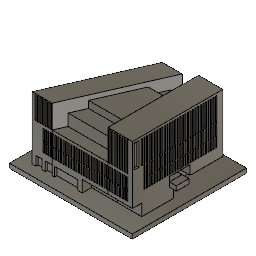
Marshgate v15 (Autodesk Fusion 360 design; units mm, degrees)
Autodesk Fusion 360 part; units mm, degrees
(part 1 of 2)
sketch "Sketch1" plane through (0, 0, 0) normal (0, 0, 1) x (1, 0, 0)
  line L0 (45.5671, 66.2073) -> (45.5671, 27.2073)
  line L1 (45.5671, 27.2073) -> (2.2671, 27.2073)
  line L2 (45.5671, 66.2073) -> (19.3671, 66.2073)
  line L3 (19.3671, 66.2073) -> (2.2671, 27.2073)
  line L4 (45.5671, 66.2073) -> (35, 66.2073)
  line L5 (35, 27.2073) -> (35, 66.2073)
  line L6 (28.0686, 66.2073) -> (10.9686, 27.2073)
  line L7 (13.0575, 31.9714) -> (35, 31.9714)
  line L8 (15.7468, 38.1049) -> (35, 38.1049)
  line L9 (23.5655, 55.9369) -> (35, 55.9369)
  line L10 (26.4855, 62.5965) -> (35, 62.5965)
  line L11 (42, 62) -> (26, 69)
  line L12 (26, 69) -> (24, 61)
  line L13 (24, 61) -> (42, 62)
  line L14 (50.0207, 22.6472) -> (-2.9555, 22.6472)
  line L15 (-2.9555, 22.6472) -> (-2.9555, 71.9468)
  line L16 (-2.9555, 71.9468) -> (50.0207, 71.9468)
  line L17 (50.0207, 71.9468) -> (50.0207, 22.6472)
  line L18 (-2.9555, 33.4173) -> (13.9382, 71.9468)
  dimension "d1" = 39
  dimension "d2" = 43.3
  dimension "d3" = 26.2
  constraint vertical L0
  constraint perpendicular L0 L1
  constraint perpendicular L0 L2
  constraint coincident L2 L4.end
  constraint coincident L1 L5.start
  constraint perpendicular L2 L5
  constraint coincident L2 L6.start
  constraint coincident L1 L6.end
  constraint parallel L3 L6
  constraint coincident L6 L7.start
  constraint coincident L5 L7.end
  constraint perpendicular L5 L7
  constraint coincident L6 L8.start
  constraint coincident L5 L8.end
  constraint perpendicular L5 L8
  constraint coincident L6 L9.start
  constraint coincident L5 L9.end
  constraint perpendicular L5 L9
  constraint coincident L6 L10.start
  constraint coincident L5 L10.end
  constraint perpendicular L5 L10
  constraint horizontal L14
  constraint vertical L15
  constraint horizontal L16
  constraint vertical L17
  constraint coincident L15 L18.start
  constraint coincident L16 L18.end
  constraint parallel L3 L18
  measures "d1" distance of L0.start L0.end
  measures "d2" distance of L0.end L1.end
  measures "d3" distance of L0.start L2.end
extrude "Extrude1" add sketch "Sketch1" along normal blind 30 contours L0 L1 L2 L4 L5 L11 L13 | L5 L11 L13 makes body 1
extrude "Extrude2" add sketch "Sketch1" along normal blind 27 separate body contours L1 L2 L3 L6 L12 L13 | L2 L6 L12 L13 makes body 2
extrude "Extrude3" add sketch "Sketch1" along normal blind 25 separate body contours L5 L6 L8 L9 makes body 3
extrude "Extrude4" add sketch "Sketch1" along normal blind 22 separate body contours L5 L6 L7 L8 makes body 4
extrude "Extrude5" add sketch "Sketch1" along normal blind 17 separate body contours L1 L5 L6 L7 makes body 5
extrude "Extrude6" add sketch "Sketch1" along normal blind 22 separate body contours L5 L6 L10 L13 | L5 L6 L9 L13 makes body 6
extrude "Extrude7" add sketch "Sketch1" along normal blind 10 separate body contours L2 L5 L11 | L2 L5 L6 L10 L11 makes body 7
sketch "Sketch2" plane through (0, 27.2073, 0) normal (0, -1, 0) x (1, 0, 0)
  line L0 (10.9686, 0) -> (35, 0)
  line L1 (35, 0) -> (35, 17)
  line L2 (35, 17) -> (10.9686, 17)
  line L3 (10.9686, 17) -> (10.9686, 0)
  line L4 (35, 10) -> (28.0686, 10)
  line L5 (2.2671, 0) -> (10.9686, 0)
  line L6 (10.9686, 0) -> (10.9686, 27)
  line L7 (10.9686, 27) -> (2.2671, 27)
  line L8 (2.2671, 27) -> (2.2671, 0)
  line L9 (35, 0) -> (45.5671, 0)
  line L10 (45.5671, 0) -> (45.5671, 30)
  line L11 (45.5671, 30) -> (35, 30)
  line L12 (35, 30) -> (35, 0)
  line L13 (2.2671, 0) -> (45.5671, 0)
  line L14 (45.5671, 0) -> (45.5671, 5.0322)
  line L15 (45.5671, 5.0322) -> (2.2671, 5.0322)
  line L16 (2.2671, 5.0322) -> (2.2671, 0)
  line L17 (23.9171, 5.0322) -> (35, 5.0322)
  line L18 (35, 5.0322) -> (35, 0)
  line L19 (35, 0) -> (23.9171, 0)
  line L20 (23.9171, 0) -> (23.9171, 5.0322)
  line L21 (22, 4) -> (12, 4)
  line L22 (12, 4) -> (12, 0)
  line L23 (12, 0) -> (22, 0)
  line L24 (22, 0) -> (22, 4)
  line L25 (4, 4) -> (6.6179, 4)
  line L26 (6.6179, 4) -> (6.6179, 0)
  line L27 (6.6179, 0) -> (4, 0)
  line L28 (4, 0) -> (4, 4)
  line L29 (8, 4) -> (10.9686, 4)
  line L30 (10.9686, 4) -> (10.9686, 0)
  line L31 (10.9686, 0) -> (8, 0)
  line L32 (8, 0) -> (8, 4)
  line L33 (24.9513, 10.7057) -> (24.4513, 10.7057)
  line L34 (27.7625, 10.7057) -> (27.7625, 15.6501)
  line L35 (23.3549, 10.3545) -> (23.8549, 10.3545)
  line L36 (26.6587, 10.7057) -> (26.6587, 15.6501)
  line L37 (24.4513, 10.7057) -> (24.4513, 15.6501)
  line L38 (17.2292, 6.6128) -> (16.7292, 6.6128)
  line L39 (17.8291, 15.6501) -> (18.3291, 15.6501)
  line L40 (18.3291, 15.6501) -> (18.3291, 10.7057)
  line L41 (21.6402, 15.6501) -> (21.6402, 10.7057)
  line L42 (17.8334, 10.3545) -> (18.3334, 10.3545)
  line L43 (20.042, 10.3545) -> (20.542, 10.3545)
  line L44 (22.2439, 15.6501) -> (22.7439, 15.6501)
  line L45 (21.1402, 10.7057) -> (21.1402, 15.6501)
  line L46 (18.9377, 10.3545) -> (19.4377, 10.3545)
  line L47 (18.9328, 15.6501) -> (19.4328, 15.6501)
  line L48 (21.1463, 10.3545) -> (21.6463, 10.3545)
  line L49 (22.7439, 10.7057) -> (22.2439, 10.7057)
  line L50 (19.4328, 10.7057) -> (18.9328, 10.7057)
  line L51 (21.6402, 10.7057) -> (21.1402, 10.7057)
  line L52 (20.0365, 15.6501) -> (20.5365, 15.6501)
  line L53 (23.8476, 15.6501) -> (23.8476, 10.7057)
  line L54 (24.4592, 10.3545) -> (24.9592, 10.3545)
  line L55 (23.3476, 15.6501) -> (23.8476, 15.6501)
  line L56 (27.1587, 10.7057) -> (26.6587, 10.7057)
  line L57 (25.5634, 10.3545) -> (26.0634, 10.3545)
  line L58 (25.555, 15.6501) -> (26.055, 15.6501)
  line L59 (23.3476, 10.7057) -> (23.3476, 15.6501)
  line L60 (12.812, 6.6128) -> (12.312, 6.6128)
  line L61 (24.9592, 6.6128) -> (24.4592, 6.6128)
  line L62 (20.542, 6.6128) -> (20.042, 6.6128)
  line L63 (21.6463, 6.6128) -> (21.1463, 6.6128)
  line L64 (26.0634, 6.6128) -> (25.5634, 6.6128)
  line L65 (18.3334, 6.6128) -> (17.8334, 6.6128)
  line L66 (23.8476, 10.7057) -> (23.3476, 10.7057)
  line L67 (26.6677, 10.3545) -> (27.1677, 10.3545)
  line L68 (26.6587, 15.6501) -> (27.1587, 15.6501)
  line L69 (26.055, 15.6501) -> (26.055, 10.7057)
  line L70 (27.1587, 15.6501) -> (27.1587, 10.7057)
  line L71 (26.055, 10.7057) -> (25.555, 10.7057)
  line L72 (24.9513, 15.6501) -> (24.9513, 10.7057)
  line L73 (24.4513, 15.6501) -> (24.9513, 15.6501)
  line L74 (25.555, 10.7057) -> (25.555, 15.6501)
  line L75 (16.1217, 15.6501) -> (16.1217, 10.7057)
  line L76 (11.2077, 10.3545) -> (11.7077, 10.3545)
  line L77 (13.9143, 15.6501) -> (13.9143, 10.7057)
  line L78 (11.7069, 15.6501) -> (11.7069, 10.7057)
  line L79 (17.2254, 15.6501) -> (17.2254, 10.7057)
  line L80 (15.6249, 10.3545) -> (16.1249, 10.3545)
  line L81 (22.7506, 6.6128) -> (22.2506, 6.6128)
  line L82 (19.4377, 6.6128) -> (18.9377, 6.6128)
  line L83 (11.7077, 6.6128) -> (11.2077, 6.6128)
  line L84 (27.1677, 6.6128) -> (26.6677, 6.6128)
  line L85 (16.1249, 6.6128) -> (15.6249, 6.6128)
  line L86 (23.8549, 6.6128) -> (23.3549, 6.6128)
  line L87 (15.0206, 6.6128) -> (14.5206, 6.6128)
  line L88 (10.6034, 6.6128) -> (10.1034, 6.6128)
  line L89 (13.9163, 6.6128) -> (13.4163, 6.6128)
  line L90 (23.3549, 6.6128) -> (23.3549, 10.3545)
  line L91 (16.1249, 10.3545) -> (16.1249, 6.6128)
  line L92 (10.6034, 10.3545) -> (10.6034, 6.6128)
  line L93 (16.7292, 6.6128) -> (16.7292, 10.3545)
  line L94 (27.772, 10.3545) -> (28.272, 10.3545)
  line L95 (15.0206, 10.3545) -> (15.0206, 6.6128)
  line L96 (24.4592, 6.6128) -> (24.4592, 10.3545)
  line L97 (27.7625, 15.6501) -> (28.2625, 15.6501)
  line L98 (22.2506, 6.6128) -> (22.2506, 10.3545)
  line L99 (26.0634, 10.3545) -> (26.0634, 6.6128)
  line L100 (28.2625, 10.7057) -> (27.7625, 10.7057)
  line L101 (21.6463, 10.3545) -> (21.6463, 6.6128)
  line L102 (22.7506, 10.3545) -> (22.7506, 6.6128)
  line L103 (20.542, 10.3545) -> (20.542, 6.6128)
  line L104 (13.4163, 6.6128) -> (13.4163, 10.3545)
  line L105 (18.9377, 6.6128) -> (18.9377, 10.3545)
  line L106 (19.4377, 10.3545) -> (19.4377, 6.6128)
  line L107 (27.772, 6.6128) -> (27.772, 10.3545)
  line L108 (25.5634, 6.6128) -> (25.5634, 10.3545)
  line L109 (18.3334, 10.3545) -> (18.3334, 6.6128)
  line L110 (21.1463, 6.6128) -> (21.1463, 10.3545)
  line L111 (20.5365, 10.7057) -> (20.0365, 10.7057)
  line L112 (20.5365, 15.6501) -> (20.5365, 10.7057)
  line L113 (18.9328, 10.7057) -> (18.9328, 15.6501)
  line L114 (22.2439, 10.7057) -> (22.2439, 15.6501)
  line L115 (18.3291, 10.7057) -> (17.8291, 10.7057)
  line L116 (21.1402, 15.6501) -> (21.6402, 15.6501)
  line L117 (20.0365, 10.7057) -> (20.0365, 15.6501)
  line L118 (19.4328, 15.6501) -> (19.4328, 10.7057)
  line L119 (22.2506, 10.3545) -> (22.7506, 10.3545)
  line L120 (22.7439, 15.6501) -> (22.7439, 10.7057)
  line L121 (17.8291, 10.7057) -> (17.8291, 15.6501)
  line L122 (13.4163, 10.3545) -> (13.9163, 10.3545)
  line L123 (16.7254, 15.6501) -> (17.2254, 15.6501)
  line L124 (16.7254, 10.7057) -> (16.7254, 15.6501)
  line L125 (12.312, 10.3545) -> (12.812, 10.3545)
  line L126 (11.2069, 15.6501) -> (11.7069, 15.6501)
  line L127 (14.5206, 10.3545) -> (15.0206, 10.3545)
  line L128 (17.2254, 10.7057) -> (16.7254, 10.7057)
  line L129 (15.018, 15.6501) -> (15.018, 10.7057)
  line L130 (13.4143, 15.6501) -> (13.9143, 15.6501)
  line L131 (13.9143, 10.7057) -> (13.4143, 10.7057)
  line L132 (11.7069, 10.7057) -> (11.2069, 10.7057)
  line L133 (10.6034, 15.6501) -> (10.6034, 10.7057)
  line L134 (16.7292, 10.3545) -> (17.2292, 10.3545)
  line L135 (12.8106, 10.7057) -> (12.3106, 10.7057)
  line L136 (16.1217, 10.7057) -> (15.6217, 10.7057)
  line L137 (14.518, 15.6501) -> (15.018, 15.6501)
  line L138 (10.1034, 10.3545) -> (10.6034, 10.3545)
  line L139 (27.1677, 10.3545) -> (27.1677, 6.6128)
  line L140 (24.9592, 10.3545) -> (24.9592, 6.6128)
  line L141 (10.1034, 6.6128) -> (10.1034, 10.3545)
  line L142 (12.812, 10.3545) -> (12.812, 6.6128)
  line L143 (11.2077, 6.6128) -> (11.2077, 10.3545)
  line L144 (11.7077, 10.3545) -> (11.7077, 6.6128)
  line L145 (26.6677, 6.6128) -> (26.6677, 10.3545)
  line L146 (15.6249, 6.6128) -> (15.6249, 10.3545)
  line L147 (23.8549, 10.3545) -> (23.8549, 6.6128)
  line L148 (20.042, 6.6128) -> (20.042, 10.3545)
  line L149 (17.8334, 6.6128) -> (17.8334, 10.3545)
  line L150 (17.2292, 10.3545) -> (17.2292, 6.6128)
  line L151 (14.5206, 6.6128) -> (14.5206, 10.3545)
  line L152 (13.9163, 10.3545) -> (13.9163, 6.6128)
  line L153 (12.312, 6.6128) -> (12.312, 10.3545)
  line L154 (11.2069, 10.7057) -> (11.2069, 15.6501)
  line L155 (10.1034, 10.7057) -> (10.1034, 15.6501)
  line L156 (15.6217, 15.6501) -> (16.1217, 15.6501)
  line L157 (15.018, 10.7057) -> (14.518, 10.7057)
  line L158 (10.6034, 10.7057) -> (10.1034, 10.7057)
  line L159 (14.518, 10.7057) -> (14.518, 15.6501)
  line L160 (12.3106, 10.7057) -> (12.3106, 15.6501)
  line L161 (13.4143, 10.7057) -> (13.4143, 15.6501)
  line L162 (10.1034, 15.6501) -> (10.6034, 15.6501)
  line L163 (15.6217, 10.7057) -> (15.6217, 15.6501)
  line L164 (12.3106, 15.6501) -> (12.8106, 15.6501)
  line L165 (12.8106, 15.6501) -> (12.8106, 10.7057)
  line L166 (38.8149, 6.6128) -> (38.8149, 10.3545)
  line L167 (31.0736, 15.6501) -> (31.5736, 15.6501)
  line L168 (36.6063, 10.3545) -> (37.1063, 10.3545)
  line L169 (31.5736, 15.6501) -> (31.5736, 10.7057)
  line L170 (32.6773, 10.7057) -> (32.1773, 10.7057)
  line L171 (37.6958, 15.6501) -> (38.1958, 15.6501)
  line L172 (35.502, 10.3545) -> (36.002, 10.3545)
  line L173 (28.8662, 15.6501) -> (29.3662, 15.6501)
  line L174 (29.9806, 10.3545) -> (30.4806, 10.3545)
  line L175 (36.002, 6.6128) -> (35.502, 6.6128)
  line L176 (32.1773, 10.7057) -> (32.1773, 15.6501)
  line L177 (29.9806, 6.6128) -> (29.9806, 10.3545)
  line L178 (41.0234, 6.6128) -> (41.0234, 10.3545)
  line L179 (28.8763, 6.6128) -> (28.8763, 10.3545)
  line L180 (39.9192, 6.6128) -> (39.9192, 10.3545)
  line L181 (30.4699, 15.6501) -> (30.4699, 10.7057)
  line L182 (31.5849, 10.3545) -> (31.5849, 6.6128)
  line L183 (34.8977, 10.3545) -> (34.8977, 6.6128)
  line L184 (36.6063, 6.6128) -> (36.6063, 10.3545)
  line L185 (39.2995, 10.7057) -> (38.7995, 10.7057)
  line L186 (39.2995, 15.6501) -> (39.2995, 10.7057)
  line L187 (33.781, 10.7057) -> (33.281, 10.7057)
  line L188 (29.3662, 10.7057) -> (28.8662, 10.7057)
  line L189 (35.4884, 15.6501) -> (35.9884, 15.6501)
  line L190 (39.9032, 15.6501) -> (40.4032, 15.6501)
  line L191 (29.3662, 15.6501) -> (29.3662, 10.7057)
  line L192 (34.8847, 15.6501) -> (34.8847, 10.7057)
  line L193 (32.1892, 10.3545) -> (32.6892, 10.3545)
  line L194 (29.9699, 15.6501) -> (30.4699, 15.6501)
  line L195 (36.5921, 10.7057) -> (36.5921, 15.6501)
  line L196 (32.1773, 15.6501) -> (32.6773, 15.6501)
  line L197 (41.5234, 6.6128) -> (41.0234, 6.6128)
  line L198 (41.0069, 10.7057) -> (41.0069, 15.6501)
  line L199 (28.272, 10.3545) -> (28.272, 6.6128)
  line L200 (33.7934, 6.6128) -> (33.2934, 6.6128)
  line L201 (41.5069, 15.6501) -> (41.5069, 10.7057)
  line L202 (36.002, 10.3545) -> (36.002, 6.6128)
  line L203 (38.8149, 10.3545) -> (39.3149, 10.3545)
  line L204 (28.8662, 10.7057) -> (28.8662, 15.6501)
  line L205 (41.5234, 10.3545) -> (41.5234, 6.6128)
  line L206 (28.2625, 15.6501) -> (28.2625, 10.7057)
  line L207 (41.5069, 10.7057) -> (41.0069, 10.7057)
  line L208 (37.7106, 6.6128) -> (37.7106, 10.3545)
  line L209 (37.6958, 10.7057) -> (37.6958, 15.6501)
  line L210 (39.9032, 10.7057) -> (39.9032, 15.6501)
  line L211 (39.3149, 6.6128) -> (38.8149, 6.6128)
  line L212 (37.0921, 15.6501) -> (37.0921, 10.7057)
  line L213 (32.6892, 10.3545) -> (32.6892, 6.6128)
  line L214 (34.8977, 6.6128) -> (34.3977, 6.6128)
  line L215 (40.4192, 6.6128) -> (39.9192, 6.6128)
  line L216 (39.3149, 10.3545) -> (39.3149, 6.6128)
  line L217 (29.9699, 10.7057) -> (29.9699, 15.6501)
  line L218 (36.5921, 15.6501) -> (37.0921, 15.6501)
  line L219 (30.4806, 10.3545) -> (30.4806, 6.6128)
  line L220 (39.9192, 10.3545) -> (40.4192, 10.3545)
  line L221 (34.3847, 10.7057) -> (34.3847, 15.6501)
  line L222 (29.3763, 10.3545) -> (29.3763, 6.6128)
  line L223 (28.8763, 10.3545) -> (29.3763, 10.3545)
  line L224 (33.281, 15.6501) -> (33.781, 15.6501)
  line L225 (29.3763, 6.6128) -> (28.8763, 6.6128)
  line L226 (31.0849, 6.6128) -> (31.0849, 10.3545)
  line L227 (31.5849, 6.6128) -> (31.0849, 6.6128)
  line L228 (32.1892, 6.6128) -> (32.1892, 10.3545)
  line L229 (37.1063, 10.3545) -> (37.1063, 6.6128)
  line L230 (34.3977, 10.3545) -> (34.8977, 10.3545)
  line L231 (37.7106, 10.3545) -> (38.2106, 10.3545)
  line L232 (33.2934, 6.6128) -> (33.2934, 10.3545)
  line L233 (38.2106, 6.6128) -> (37.7106, 6.6128)
  line L234 (38.1958, 10.7057) -> (37.6958, 10.7057)
  line L235 (38.7995, 10.7057) -> (38.7995, 15.6501)
  line L236 (31.5736, 10.7057) -> (31.0736, 10.7057)
  line L237 (30.4699, 10.7057) -> (29.9699, 10.7057)
  line L238 (31.0736, 10.7057) -> (31.0736, 15.6501)
  line L239 (32.6773, 15.6501) -> (32.6773, 10.7057)
  line L240 (33.281, 10.7057) -> (33.281, 15.6501)
  line L241 (28.272, 6.6128) -> (27.772, 6.6128)
  line L242 (35.4884, 10.7057) -> (35.4884, 15.6501)
  line L243 (33.2934, 10.3545) -> (33.7934, 10.3545)
  line L244 (37.1063, 6.6128) -> (36.6063, 6.6128)
  line L245 (33.781, 15.6501) -> (33.781, 10.7057)
  line L246 (41.0234, 10.3545) -> (41.5234, 10.3545)
  line L247 (35.9884, 15.6501) -> (35.9884, 10.7057)
  line L248 (37.0921, 10.7057) -> (36.5921, 10.7057)
  line L249 (33.7934, 10.3545) -> (33.7934, 6.6128)
  line L250 (35.502, 6.6128) -> (35.502, 10.3545)
  line L251 (41.0069, 15.6501) -> (41.5069, 15.6501)
  line L252 (31.0849, 10.3545) -> (31.5849, 10.3545)
  line L253 (40.4192, 10.3545) -> (40.4192, 6.6128)
  line L254 (35.9884, 10.7057) -> (35.4884, 10.7057)
  line L255 (38.1958, 15.6501) -> (38.1958, 10.7057)
  line L256 (38.2106, 10.3545) -> (38.2106, 6.6128)
  line L257 (40.4032, 10.7057) -> (39.9032, 10.7057)
  line L258 (38.7995, 15.6501) -> (39.2995, 15.6501)
  line L259 (30.4806, 6.6128) -> (29.9806, 6.6128)
  line L260 (34.3977, 6.6128) -> (34.3977, 10.3545)
  line L261 (34.8847, 10.7057) -> (34.3847, 10.7057)
  line L262 (34.3847, 15.6501) -> (34.8847, 15.6501)
  line L263 (40.4032, 15.6501) -> (40.4032, 10.7057)
  line L264 (32.6892, 6.6128) -> (32.1892, 6.6128)
  line L265 (42.5069, 15.6501) -> (42.5069, 10.7057)
  line L266 (42.5069, 10.7057) -> (42.0069, 10.7057)
  line L267 (42.0069, 10.7057) -> (42.0069, 15.6501)
  line L268 (42.0069, 15.6501) -> (42.5069, 15.6501)
  line L269 (42.5234, 10.3545) -> (42.5234, 6.6128)
  line L270 (42.0234, 6.6128) -> (42.0234, 10.3545)
  line L271 (42.0234, 10.3545) -> (42.5234, 10.3545)
  line L272 (42.5234, 6.6128) -> (42.0234, 6.6128)
  line L273 (43.5069, 15.6501) -> (43.5069, 10.7057)
  line L274 (43.5069, 10.7057) -> (43.0069, 10.7057)
  line L275 (43.0069, 10.7057) -> (43.0069, 15.6501)
  line L276 (43.0069, 15.6501) -> (43.5069, 15.6501)
  line L277 (43.5234, 10.3545) -> (43.5234, 6.6128)
  line L278 (43.0234, 6.6128) -> (43.0234, 10.3545)
  line L279 (43.0234, 10.3545) -> (43.5234, 10.3545)
  line L280 (43.5234, 6.6128) -> (43.0234, 6.6128)
  line L281 (9.5069, 15.6501) -> (9.5069, 10.7057)
  line L282 (9.5069, 10.7057) -> (9.0069, 10.7057)
  line L283 (9.0069, 10.7057) -> (9.0069, 15.6501)
  line L284 (9.0069, 15.6501) -> (9.5069, 15.6501)
  line L285 (9.5234, 10.3545) -> (9.5234, 6.6128)
  line L286 (9.0234, 6.6128) -> (9.0234, 10.3545)
  line L287 (9.0234, 10.3545) -> (9.5234, 10.3545)
  line L288 (9.5234, 6.6128) -> (9.0234, 6.6128)
  line L289 (8.5234, 10.3545) -> (8.5234, 6.6128)
  line L290 (8.0234, 6.6128) -> (8.0234, 10.3545)
  line L291 (8.0234, 10.3545) -> (8.5234, 10.3545)
  line L292 (8.5234, 6.6128) -> (8.0234, 6.6128)
  line L293 (8.5069, 10.7057) -> (8.0069, 10.7057)
  line L294 (8.0069, 10.7057) -> (8.0069, 15.6501)
  line L295 (8.5069, 15.6501) -> (8.5069, 10.7057)
  line L296 (8.0069, 15.6501) -> (8.5069, 15.6501)
  line L297 (7.5234, 10.3545) -> (7.5234, 6.6128)
  line L298 (7.0234, 6.6128) -> (7.0234, 10.3545)
  line L299 (7.0234, 10.3545) -> (7.5234, 10.3545)
  line L300 (7.5234, 6.6128) -> (7.0234, 6.6128)
  line L301 (7.5069, 10.7057) -> (7.0069, 10.7057)
  line L302 (7.0069, 10.7057) -> (7.0069, 15.6501)
  line L303 (7.5069, 15.6501) -> (7.5069, 10.7057)
  line L304 (7.0069, 15.6501) -> (7.5069, 15.6501)
  line L305 (35.4884, 29.481) -> (35.9884, 29.481)
  line L306 (35.9884, 29.481) -> (35.9884, 16.9429)
  line L307 (35.9884, 16.9429) -> (35.4884, 16.9429)
  line L308 (35.4884, 16.9429) -> (35.4884, 29.481)
  line L309 (37.0669, 29.481) -> (37.0669, 16.9429)
  line L310 (36.5669, 16.9429) -> (36.5669, 29.481)
  line L311 (36.5669, 29.481) -> (37.0669, 29.481)
  line L312 (37.0669, 16.9429) -> (36.5669, 16.9429)
  line L313 (38.1455, 29.481) -> (38.1455, 16.9429)
  line L314 (37.6455, 16.9429) -> (37.6455, 29.481)
  line L315 (37.6455, 29.481) -> (38.1455, 29.481)
  line L316 (38.1455, 16.9429) -> (37.6455, 16.9429)
  line L317 (39.2241, 29.481) -> (39.2241, 16.9429)
  line L318 (38.7241, 16.9429) -> (38.7241, 29.481)
  line L319 (38.7241, 29.481) -> (39.2241, 29.481)
  line L320 (39.2241, 16.9429) -> (38.7241, 16.9429)
  line L321 (40.3027, 29.481) -> (40.3027, 16.9429)
  line L322 (39.8027, 16.9429) -> (39.8027, 29.481)
  line L323 (39.8027, 29.481) -> (40.3027, 29.481)
  line L324 (40.3027, 16.9429) -> (39.8027, 16.9429)
  line L325 (41.3812, 29.481) -> (41.3812, 16.9429)
  line L326 (40.8812, 16.9429) -> (40.8812, 29.481)
  line L327 (40.8812, 29.481) -> (41.3812, 29.481)
  line L328 (41.3812, 16.9429) -> (40.8812, 16.9429)
  line L329 (42.4598, 29.481) -> (42.4598, 16.9429)
  line L330 (41.9598, 16.9429) -> (41.9598, 29.481)
  line L331 (41.9598, 29.481) -> (42.4598, 29.481)
  line L332 (42.4598, 16.9429) -> (41.9598, 16.9429)
  line L333 (43.5384, 29.481) -> (43.5384, 16.9429)
  line L334 (43.0384, 16.9429) -> (43.0384, 29.481)
  line L335 (43.0384, 29.481) -> (43.5384, 29.481)
  line L336 (43.5384, 16.9429) -> (43.0384, 16.9429)
  line L337 (38.7241, 16.9429) -> (38.7241, 29.481)
  line L338 (41.9598, 16.9429) -> (41.9598, 29.481)
  line L339 (43.0384, 16.9429) -> (43.0384, 29.481)
  line L340 (37.6455, 16.9429) -> (37.6455, 29.481)
  line L341 (38.1455, 29.481) -> (38.1455, 16.9429)
  line L342 (37.0669, 29.481) -> (37.0669, 16.9429)
  line L343 (41.3812, 29.481) -> (41.3812, 16.9429)
  line L344 (35.4884, 16.9429) -> (35.4884, 29.481)
  line L345 (39.2241, 29.481) -> (39.2241, 16.9429)
  line L346 (43.5384, 29.481) -> (43.5384, 16.9429)
  line L347 (40.3027, 29.481) -> (40.3027, 16.9429)
  line L348 (42.4598, 29.481) -> (42.4598, 16.9429)
  line L349 (35.9884, 29.481) -> (35.9884, 16.9429)
  line L350 (40.8812, 16.9429) -> (40.8812, 29.481)
  line L351 (39.8027, 16.9429) -> (39.8027, 29.481)
  line L352 (36.5669, 16.9429) -> (36.5669, 29.481)
  line L353 (10.0384, 26.4977) -> (10.5384, 26.4977)
  line L354 (8.3812, 16.9429) -> (7.8812, 16.9429)
  line L355 (10.5384, 26.4977) -> (10.5384, 16.9429)
  line L356 (10.0384, 16.9429) -> (10.0384, 26.4977)
  line L357 (9.4598, 16.9429) -> (8.9598, 16.9429)
  line L358 (8.3812, 26.4977) -> (8.3812, 16.9429)
  line L359 (10.5384, 16.9429) -> (10.0384, 16.9429)
  line L360 (8.9598, 26.4977) -> (9.4598, 26.4977)
  line L361 (9.4598, 26.4977) -> (9.4598, 16.9429)
  line L362 (7.8812, 26.4977) -> (8.3812, 26.4977)
  line L363 (7.8812, 16.9429) -> (7.8812, 26.4977)
  line L364 (8.3812, 29.481) -> (8.3812, 16.9429)
  line L365 (8.9598, 16.9429) -> (8.9598, 29.481)
  line L366 (5.1455, 26.4977) -> (5.1455, 16.9429)
  line L367 (2.9884, 26.4977) -> (2.9884, 16.9429)
  line L368 (7.8812, 16.9429) -> (7.8812, 29.481)
  line L369 (7.3027, 26.4977) -> (7.3027, 16.9429)
  line L370 (2.4884, 16.9429) -> (2.4884, 26.4977)
  line L371 (2.9884, 16.9429) -> (2.4884, 16.9429)
  line L372 (4.0669, 16.9429) -> (3.5669, 16.9429)
  line L373 (7.3027, 29.481) -> (7.3027, 16.9429)
  line L374 (3.5669, 26.4977) -> (4.0669, 26.4977)
  line L375 (10.5384, 29.481) -> (10.5384, 16.9429)
  line L376 (5.7241, 16.9429) -> (5.7241, 26.4977)
  line L377 (3.5669, 16.9429) -> (3.5669, 26.4977)
  line L378 (10.0384, 16.9429) -> (10.0384, 29.481)
  line L379 (6.8027, 26.4977) -> (7.3027, 26.4977)
  line L380 (4.6455, 26.4977) -> (5.1455, 26.4977)
  line L381 (4.0669, 26.4977) -> (4.0669, 16.9429)
  line L382 (2.4884, 26.4977) -> (2.9884, 26.4977)
  line L383 (6.8027, 16.9429) -> (6.8027, 26.4977)
  line L384 (6.2241, 16.9429) -> (5.7241, 16.9429)
  line L385 (6.2241, 26.4977) -> (6.2241, 16.9429)
  line L386 (8.9598, 16.9429) -> (8.9598, 26.4977)
  line L387 (9.4598, 29.481) -> (9.4598, 16.9429)
  line L388 (5.7241, 16.9429) -> (5.7241, 29.481)
  line L389 (6.2241, 29.481) -> (6.2241, 16.9429)
  line L390 (5.1455, 29.481) -> (5.1455, 16.9429)
  line L391 (7.3027, 16.9429) -> (6.8027, 16.9429)
  line L392 (5.1455, 16.9429) -> (4.6455, 16.9429)
  line L393 (4.6455, 16.9429) -> (4.6455, 26.4977)
  line L394 (5.7241, 26.4977) -> (6.2241, 26.4977)
  line L395 (4.6455, 16.9429) -> (4.6455, 29.481)
  line L396 (3.5669, 16.9429) -> (3.5669, 26.3979)
  line L397 (2.4884, 16.9429) -> (2.4884, 29.481)
  line L398 (6.8027, 16.9429) -> (6.8027, 29.481)
  line L399 (4.0669, 26.3348) -> (4.0669, 16.9429)
  line L400 (2.9884, 29.481) -> (2.9884, 16.9429)
  point P0 (45.5671, 0)
  point P1 (31.569, 16)
  point P2 (37.0862, 16)
  point P3 (37.6897, 16)
  point P4 (38.1897, 16)
  point P5 (38.7931, 16)
  point P6 (33.2759, 16)
  point P7 (33.7759, 16)
  point P8 (29.9655, 16)
  point P9 (27.7586, 16)
  point P10 (31.069, 16)
  point P11 (27.1552, 16)
  point P12 (26.6552, 16)
  point P13 (29.3621, 16)
  point P14 (28.8621, 16)
  point P15 (34.3793, 16)
  point P16 (34.8793, 16)
  point P17 (35.9828, 16)
  point P18 (28.2586, 16)
  point P19 (32.6724, 16)
  point P20 (30.4655, 16)
  point P21 (32.1724, 16)
  point P22 (35.4828, 16)
  point P23 (36.5862, 16)
  point P24 (41, 16)
  point P25 (40.3966, 16)
  point P26 (39.2931, 16)
  point P27 (41.5, 16)
  point P28 (39.8966, 16)
  point P29 (30, 6)
  point P30 (21.0949, 6)
  point P31 (8, 16)
  point P32 (9.5, 16)
  point P33 (9, 16)
  point P34 (22.7414, 16)
  point P35 (23.3448, 16)
  point P36 (23.8448, 16)
  point P37 (24.4483, 16)
  point P38 (25.5517, 16)
  point P39 (26.0517, 16)
  point P40 (24.9483, 16)
  point P41 (14.5172, 16)
  point P42 (11.2069, 16)
  point P43 (16.1207, 16)
  point P44 (17.2241, 16)
  point P45 (11.7069, 16)
  point P46 (12.3103, 16)
  point P47 (18.3276, 16)
  point P48 (21.6379, 16)
  point P49 (15.0172, 16)
  point P50 (10.1034, 16)
  point P51 (10.6034, 16)
  point P52 (12.8103, 16)
  point P53 (13.4138, 16)
  point P54 (13.9138, 16)
  point P55 (15.6207, 16)
  point P56 (16.7241, 16)
  point P57 (17.8276, 16)
  point P58 (18.931, 16)
  point P59 (19.431, 16)
  point P60 (20.0345, 16)
  point P61 (20.5345, 16)
  point P62 (21.1379, 16)
  point P63 (22.2414, 16)
  point P64 (2, 17)
  point P65 (12.5671, 30)
  point P66 (2, 30)
  dimension "d120" = 29.8
  dimension "d121" = 0
  dimension "d124" = 30.92
  dimension "d125" = 0
  dimension "d126" = 0.5
  dimension "d127" = 0.5
  dimension "d130" = 7.55
  dimension "d131" = 0
  dimension "d132" = 0.5
  dimension "d135" = 7.55
  dimension "d136" = 0
  dimension "d137" = 0.5
  dimension "d138" = 0.5
  constraint horizontal L13
  constraint vertical L14
  constraint horizontal L15
  constraint vertical L16
  constraint coincident L10 L14.end
  constraint coincident L5.start L8.end
  constraint horizontal L17
  constraint vertical L18
  constraint horizontal L19
  constraint vertical L20
  constraint coincident L0.end L1.start
  constraint midpoint L15 L17.start
  constraint horizontal L21
  constraint vertical L22
  constraint horizontal L23
  constraint vertical L24
  constraint coincident L0 L22.end
  constraint horizontal L25
  constraint vertical L26
  constraint horizontal L27
  constraint vertical L28
  constraint midpoint L5 L26.end
  constraint horizontal L29
  constraint vertical L30
  constraint horizontal L31
  constraint vertical L32
  constraint coincident L0.start L3.end
  constraint horizontal L162
  constraint vertical L133
  constraint horizontal L158
  constraint vertical L155
  constraint horizontal L126
  constraint vertical L78
  constraint horizontal L132
  constraint vertical L154
  constraint horizontal L138
  constraint vertical L92
  constraint horizontal L88
  constraint vertical L141
  constraint horizontal L305
  constraint vertical L306
  constraint horizontal L307
  constraint vertical L308
  constraint vertical L349
  constraint vertical L344
  constraint horizontal L382
  constraint vertical L367
  constraint horizontal L371
  constraint vertical L370
  constraint vertical L400
  constraint vertical L397
  constraint coincident L396.end L377
  constraint perpendicular L7 L396
  constraint coincident L399.start L381
  constraint perpendicular L7 L399
  measures "d126" distance of L155.end L133.start
  measures "d127" distance of L305.start L305.end
  measures "d132" distance of L305.start L305.end
  measures "d137" distance of L370.end L367.start
  measures "d138" distance of L397.end L400.start
extrude "Extrude8" cut sketch "Sketch2" against normal blind 4 contours L0 L1 L12 L13 L15 L17 L18 L19 L20 | L1 L9 L10 L12 L13 L14 L15 L18 bodies 1 5
sketch "Sketch3" plane through (45.5671, 0, 0) normal (1, 0, 0) x (0, 1, 0)
  line L0 (31.2073, 5.0322) -> (31.2073, 0)
  line L1 (31.2073, 0) -> (66.2073, 0)
  line L2 (66.2073, 0) -> (66.2073, 30)
  line L3 (66.2073, 30) -> (27.2073, 30)
  line L4 (27.2073, 30) -> (27.2073, 5.0322)
  line L5 (27.2073, 5.0322) -> (31.2073, 5.0322)
  line L6 (27.2073, 5.0322) -> (66.2073, 5.0322)
  line L7 (66.2073, 5.0322) -> (66.2073, 0)
  line L8 (66.2073, 0) -> (27.2073, 0)
  line L9 (27.2073, 0) -> (27.2073, 5.0322)
  line L10 (44.8205, 5.0322) -> (27.2073, 5.0322)
  line L11 (27.2073, 5.0322) -> (27.2073, 0)
  line L12 (27.2073, 0) -> (44.8205, 0)
  line L13 (44.8205, 0) -> (44.8205, 5.0322)
  line L14 (43.0949, 5.0322) -> (52, 5.0322)
  line L15 (52, 5.0322) -> (52, 9)
  line L16 (52, 9) -> (43.0949, 9)
  line L17 (43.0949, 9) -> (43.0949, 5.0322)
  line L18 (43.0949, 7.0161) -> (48.5441, 7.0161)
  line L19 (48.5441, 7.0161) -> (48.5441, 5.0161)
  line L20 (48.5441, 5.0161) -> (43.0949, 5.0161)
  line L21 (43.0949, 5.0161) -> (43.0949, 7.0161)
  line L22 (28, 29) -> (30, 29)
  line L23 (30, 29) -> (30, 19)
  line L24 (30, 19) -> (28, 19)
  line L25 (28, 19) -> (28, 29)
  line L26 (31, 29) -> (31.5, 29)
  line L27 (31.5, 29) -> (31.5, 19)
  line L28 (31.5, 19) -> (31, 19)
  line L29 (31, 19) -> (31, 29)
  line L30 (32.1034, 19) -> (32.1034, 29)
  line L31 (32.6034, 29) -> (32.6034, 19)
  line L32 (32.1034, 29) -> (32.6034, 29)
  line L33 (32.6034, 19) -> (32.1034, 19)
  line L34 (33.2069, 19) -> (33.2069, 29)
  line L35 (33.7069, 29) -> (33.7069, 19)
  line L36 (33.2069, 29) -> (33.7069, 29)
  line L37 (33.7069, 19) -> (33.2069, 19)
  line L38 (34.3103, 19) -> (34.3103, 29)
  line L39 (34.8103, 29) -> (34.8103, 19)
  line L40 (34.3103, 29) -> (34.8103, 29)
  line L41 (34.8103, 19) -> (34.3103, 19)
  line L42 (35.4138, 19) -> (35.4138, 29)
  line L43 (35.9138, 29) -> (35.9138, 19)
  line L44 (35.4138, 29) -> (35.9138, 29)
  line L45 (35.9138, 19) -> (35.4138, 19)
  line L46 (36.5172, 19) -> (36.5172, 29)
  line L47 (37.0172, 29) -> (37.0172, 19)
  line L48 (36.5172, 29) -> (37.0172, 29)
  line L49 (37.0172, 19) -> (36.5172, 19)
  line L50 (37.6207, 19) -> (37.6207, 29)
  line L51 (38.1207, 29) -> (38.1207, 19)
  line L52 (37.6207, 29) -> (38.1207, 29)
  line L53 (38.1207, 19) -> (37.6207, 19)
  line L54 (38.7241, 19) -> (38.7241, 29)
  line L55 (39.2241, 29) -> (39.2241, 19)
  line L56 (38.7241, 29) -> (39.2241, 29)
  line L57 (39.2241, 19) -> (38.7241, 19)
  line L58 (39.8276, 19) -> (39.8276, 29)
  line L59 (40.3276, 29) -> (40.3276, 19)
  line L60 (39.8276, 29) -> (40.3276, 29)
  line L61 (40.3276, 19) -> (39.8276, 19)
  line L62 (40.931, 19) -> (40.931, 29)
  line L63 (41.431, 29) -> (41.431, 19)
  line L64 (40.931, 29) -> (41.431, 29)
  line L65 (41.431, 19) -> (40.931, 19)
  line L66 (42.0345, 19) -> (42.0345, 29)
  line L67 (42.5345, 29) -> (42.5345, 19)
  line L68 (42.0345, 29) -> (42.5345, 29)
  line L69 (42.5345, 19) -> (42.0345, 19)
  line L70 (43.1379, 19) -> (43.1379, 29)
  line L71 (43.6379, 29) -> (43.6379, 19)
  line L72 (43.1379, 29) -> (43.6379, 29)
  line L73 (43.6379, 19) -> (43.1379, 19)
  line L74 (44.2414, 19) -> (44.2414, 29)
  line L75 (44.7414, 29) -> (44.7414, 19)
  line L76 (44.2414, 29) -> (44.7414, 29)
  line L77 (44.7414, 19) -> (44.2414, 19)
  line L78 (45.3448, 19) -> (45.3448, 29)
  line L79 (45.8448, 29) -> (45.8448, 19)
  line L80 (45.3448, 29) -> (45.8448, 29)
  line L81 (45.8448, 19) -> (45.3448, 19)
  line L82 (46.4483, 19) -> (46.4483, 29)
  line L83 (46.9483, 29) -> (46.9483, 19)
  line L84 (46.4483, 29) -> (46.9483, 29)
  line L85 (46.9483, 19) -> (46.4483, 19)
  line L86 (47.5517, 19) -> (47.5517, 29)
  line L87 (48.0517, 29) -> (48.0517, 19)
  line L88 (47.5517, 29) -> (48.0517, 29)
  line L89 (48.0517, 19) -> (47.5517, 19)
  line L90 (48.6552, 19) -> (48.6552, 29)
  line L91 (49.1552, 29) -> (49.1552, 19)
  line L92 (48.6552, 29) -> (49.1552, 29)
  line L93 (49.1552, 19) -> (48.6552, 19)
  line L94 (49.7586, 19) -> (49.7586, 29)
  line L95 (50.2586, 29) -> (50.2586, 19)
  line L96 (49.7586, 29) -> (50.2586, 29)
  line L97 (50.2586, 19) -> (49.7586, 19)
  line L98 (50.8621, 19) -> (50.8621, 29)
  line L99 (51.3621, 29) -> (51.3621, 19)
  line L100 (50.8621, 29) -> (51.3621, 29)
  line L101 (51.3621, 19) -> (50.8621, 19)
  line L102 (51.9655, 19) -> (51.9655, 29)
  line L103 (52.4655, 29) -> (52.4655, 19)
  line L104 (51.9655, 29) -> (52.4655, 29)
  line L105 (52.4655, 19) -> (51.9655, 19)
  line L106 (53.069, 19) -> (53.069, 29)
  line L107 (53.569, 29) -> (53.569, 19)
  line L108 (53.069, 29) -> (53.569, 29)
  line L109 (53.569, 19) -> (53.069, 19)
  line L110 (54.1724, 19) -> (54.1724, 29)
  line L111 (54.6724, 29) -> (54.6724, 19)
  line L112 (54.1724, 29) -> (54.6724, 29)
  line L113 (54.6724, 19) -> (54.1724, 19)
  line L114 (55.2759, 19) -> (55.2759, 29)
  line L115 (55.7759, 29) -> (55.7759, 19)
  line L116 (55.2759, 29) -> (55.7759, 29)
  line L117 (55.7759, 19) -> (55.2759, 19)
  line L118 (56.3793, 19) -> (56.3793, 29)
  line L119 (56.8793, 29) -> (56.8793, 19)
  line L120 (56.3793, 29) -> (56.8793, 29)
  line L121 (56.8793, 19) -> (56.3793, 19)
  line L122 (57.4828, 19) -> (57.4828, 29)
  line L123 (57.9828, 29) -> (57.9828, 19)
  line L124 (57.4828, 29) -> (57.9828, 29)
  line L125 (57.9828, 19) -> (57.4828, 19)
  line L126 (58.5862, 19) -> (58.5862, 29)
  line L127 (59.0862, 29) -> (59.0862, 19)
  line L128 (58.5862, 29) -> (59.0862, 29)
  line L129 (59.0862, 19) -> (58.5862, 19)
  line L130 (59.6897, 19) -> (59.6897, 29)
  line L131 (60.1897, 29) -> (60.1897, 19)
  line L132 (59.6897, 29) -> (60.1897, 29)
  line L133 (60.1897, 19) -> (59.6897, 19)
  line L134 (60.7931, 19) -> (60.7931, 29)
  line L135 (61.2931, 29) -> (61.2931, 19)
  line L136 (60.7931, 29) -> (61.2931, 29)
  line L137 (61.2931, 19) -> (60.7931, 19)
  line L138 (61.8966, 19) -> (61.8966, 29)
  line L139 (62.3966, 29) -> (62.3966, 19)
  line L140 (61.8966, 29) -> (62.3966, 29)
  line L141 (62.3966, 19) -> (61.8966, 19)
  line L142 (63, 19) -> (63, 29)
  line L143 (63.5, 29) -> (63.5, 19)
  line L144 (63, 29) -> (63.5, 29)
  line L145 (63.5, 19) -> (63, 19)
  line L146 (32.1034, 18.6501) -> (32.6034, 18.6501)
  line L147 (32.6034, 18.6501) -> (32.6034, 13.7057)
  line L148 (32.6034, 13.7057) -> (32.1034, 13.7057)
  line L149 (32.1034, 13.7057) -> (32.1034, 18.6501)
  line L150 (33.2069, 18.6501) -> (33.7069, 18.6501)
  line L151 (33.7069, 18.6501) -> (33.7069, 13.7057)
  line L152 (33.7069, 13.7057) -> (33.2069, 13.7057)
  line L153 (33.2069, 13.7057) -> (33.2069, 18.6501)
  line L154 (34.3106, 13.7057) -> (34.3106, 18.6501)
  line L155 (34.8106, 18.6501) -> (34.8106, 13.7057)
  line L156 (34.3106, 18.6501) -> (34.8106, 18.6501)
  line L157 (34.8106, 13.7057) -> (34.3106, 13.7057)
  line L158 (35.4143, 13.7057) -> (35.4143, 18.6501)
  line L159 (35.9143, 18.6501) -> (35.9143, 13.7057)
  line L160 (35.4143, 18.6501) -> (35.9143, 18.6501)
  line L161 (35.9143, 13.7057) -> (35.4143, 13.7057)
  line L162 (36.518, 13.7057) -> (36.518, 18.6501)
  line L163 (37.018, 18.6501) -> (37.018, 13.7057)
  line L164 (36.518, 18.6501) -> (37.018, 18.6501)
  line L165 (37.018, 13.7057) -> (36.518, 13.7057)
  line L166 (37.6217, 13.7057) -> (37.6217, 18.6501)
  line L167 (38.1217, 18.6501) -> (38.1217, 13.7057)
  line L168 (37.6217, 18.6501) -> (38.1217, 18.6501)
  line L169 (38.1217, 13.7057) -> (37.6217, 13.7057)
  line L170 (38.7254, 13.7057) -> (38.7254, 18.6501)
  line L171 (39.2254, 18.6501) -> (39.2254, 13.7057)
  line L172 (38.7254, 18.6501) -> (39.2254, 18.6501)
  line L173 (39.2254, 13.7057) -> (38.7254, 13.7057)
  line L174 (39.8291, 13.7057) -> (39.8291, 18.6501)
  line L175 (40.3291, 18.6501) -> (40.3291, 13.7057)
  line L176 (39.8291, 18.6501) -> (40.3291, 18.6501)
  line L177 (40.3291, 13.7057) -> (39.8291, 13.7057)
  line L178 (40.9328, 13.7057) -> (40.9328, 18.6501)
  line L179 (41.4328, 18.6501) -> (41.4328, 13.7057)
  line L180 (40.9328, 18.6501) -> (41.4328, 18.6501)
  line L181 (41.4328, 13.7057) -> (40.9328, 13.7057)
  line L182 (42.0365, 13.7057) -> (42.0365, 18.6501)
  line L183 (42.5365, 18.6501) -> (42.5365, 13.7057)
  line L184 (42.0365, 18.6501) -> (42.5365, 18.6501)
  line L185 (42.5365, 13.7057) -> (42.0365, 13.7057)
  line L186 (43.1402, 13.7057) -> (43.1402, 18.6501)
  line L187 (43.6402, 18.6501) -> (43.6402, 13.7057)
  line L188 (43.1402, 18.6501) -> (43.6402, 18.6501)
  line L189 (43.6402, 13.7057) -> (43.1402, 13.7057)
  line L190 (44.2439, 13.7057) -> (44.2439, 18.6501)
  line L191 (44.7439, 18.6501) -> (44.7439, 13.7057)
  line L192 (44.2439, 18.6501) -> (44.7439, 18.6501)
  line L193 (44.7439, 13.7057) -> (44.2439, 13.7057)
  line L194 (45.3476, 13.7057) -> (45.3476, 18.6501)
  line L195 (45.8476, 18.6501) -> (45.8476, 13.7057)
  line L196 (45.3476, 18.6501) -> (45.8476, 18.6501)
  line L197 (45.8476, 13.7057) -> (45.3476, 13.7057)
  line L198 (46.4513, 13.7057) -> (46.4513, 18.6501)
  line L199 (46.9513, 18.6501) -> (46.9513, 13.7057)
  line L200 (46.4513, 18.6501) -> (46.9513, 18.6501)
  line L201 (46.9513, 13.7057) -> (46.4513, 13.7057)
  line L202 (47.555, 13.7057) -> (47.555, 18.6501)
  line L203 (48.055, 18.6501) -> (48.055, 13.7057)
  line L204 (47.555, 18.6501) -> (48.055, 18.6501)
  line L205 (48.055, 13.7057) -> (47.555, 13.7057)
  line L206 (48.6587, 13.7057) -> (48.6587, 18.6501)
  line L207 (49.1587, 18.6501) -> (49.1587, 13.7057)
  line L208 (48.6587, 18.6501) -> (49.1587, 18.6501)
  line L209 (49.1587, 13.7057) -> (48.6587, 13.7057)
  line L210 (49.7625, 13.7057) -> (49.7625, 18.6501)
  line L211 (50.2625, 18.6501) -> (50.2625, 13.7057)
  line L212 (49.7625, 18.6501) -> (50.2625, 18.6501)
  line L213 (50.2625, 13.7057) -> (49.7625, 13.7057)
  line L214 (50.8662, 13.7057) -> (50.8662, 18.6501)
  line L215 (51.3662, 18.6501) -> (51.3662, 13.7057)
  line L216 (50.8662, 18.6501) -> (51.3662, 18.6501)
  line L217 (51.3662, 13.7057) -> (50.8662, 13.7057)
  line L218 (51.9699, 13.7057) -> (51.9699, 18.6501)
  line L219 (52.4699, 18.6501) -> (52.4699, 13.7057)
  line L220 (51.9699, 18.6501) -> (52.4699, 18.6501)
  line L221 (52.4699, 13.7057) -> (51.9699, 13.7057)
  line L222 (53.0736, 13.7057) -> (53.0736, 18.6501)
  line L223 (53.5736, 18.6501) -> (53.5736, 13.7057)
  line L224 (53.0736, 18.6501) -> (53.5736, 18.6501)
  line L225 (53.5736, 13.7057) -> (53.0736, 13.7057)
  line L226 (54.1773, 13.7057) -> (54.1773, 18.6501)
  line L227 (54.6773, 18.6501) -> (54.6773, 13.7057)
  line L228 (54.1773, 18.6501) -> (54.6773, 18.6501)
  line L229 (54.6773, 13.7057) -> (54.1773, 13.7057)
  line L230 (55.281, 13.7057) -> (55.281, 18.6501)
  line L231 (55.781, 18.6501) -> (55.781, 13.7057)
  line L232 (55.281, 18.6501) -> (55.781, 18.6501)
  line L233 (55.781, 13.7057) -> (55.281, 13.7057)
  line L234 (56.3847, 13.7057) -> (56.3847, 18.6501)
  line L235 (56.8847, 18.6501) -> (56.8847, 13.7057)
  line L236 (56.3847, 18.6501) -> (56.8847, 18.6501)
  line L237 (56.8847, 13.7057) -> (56.3847, 13.7057)
  line L238 (57.4884, 13.7057) -> (57.4884, 18.6501)
  line L239 (57.9884, 18.6501) -> (57.9884, 13.7057)
  line L240 (57.4884, 18.6501) -> (57.9884, 18.6501)
  line L241 (57.9884, 13.7057) -> (57.4884, 13.7057)
  line L242 (58.5921, 13.7057) -> (58.5921, 18.6501)
  line L243 (59.0921, 18.6501) -> (59.0921, 13.7057)
  line L244 (58.5921, 18.6501) -> (59.0921, 18.6501)
  line L245 (59.0921, 13.7057) -> (58.5921, 13.7057)
  line L246 (59.6958, 13.7057) -> (59.6958, 18.6501)
  line L247 (60.1958, 18.6501) -> (60.1958, 13.7057)
  line L248 (59.6958, 18.6501) -> (60.1958, 18.6501)
  line L249 (60.1958, 13.7057) -> (59.6958, 13.7057)
  line L250 (60.7995, 13.7057) -> (60.7995, 18.6501)
  line L251 (61.2995, 18.6501) -> (61.2995, 13.7057)
  line L252 (60.7995, 18.6501) -> (61.2995, 18.6501)
  line L253 (61.2995, 13.7057) -> (60.7995, 13.7057)
  line L254 (61.9032, 13.7057) -> (61.9032, 18.6501)
  line L255 (62.4032, 18.6501) -> (62.4032, 13.7057)
  line L256 (61.9032, 18.6501) -> (62.4032, 18.6501)
  line L257 (62.4032, 13.7057) -> (61.9032, 13.7057)
  line L258 (63.0069, 13.7057) -> (63.0069, 18.6501)
  line L259 (63.5069, 18.6501) -> (63.5069, 13.7057)
  line L260 (63.0069, 18.6501) -> (63.5069, 18.6501)
  line L261 (63.5069, 13.7057) -> (63.0069, 13.7057)
  line L262 (32.1034, 13.3545) -> (32.6034, 13.3545)
  line L263 (32.6034, 13.3545) -> (32.6034, 9.6128)
  line L264 (32.6034, 9.6128) -> (32.1034, 9.6128)
  line L265 (32.1034, 9.6128) -> (32.1034, 13.3545)
  line L266 (33.7077, 13.3545) -> (33.7077, 9.6128)
  line L267 (33.2077, 9.6128) -> (33.2077, 13.3545)
  line L268 (33.2077, 13.3545) -> (33.7077, 13.3545)
  line L269 (33.7077, 9.6128) -> (33.2077, 9.6128)
  line L270 (34.812, 13.3545) -> (34.812, 9.6128)
  line L271 (34.312, 9.6128) -> (34.312, 13.3545)
  line L272 (34.312, 13.3545) -> (34.812, 13.3545)
  line L273 (34.812, 9.6128) -> (34.312, 9.6128)
  line L274 (35.9163, 13.3545) -> (35.9163, 9.6128)
  line L275 (35.4163, 9.6128) -> (35.4163, 13.3545)
  line L276 (35.4163, 13.3545) -> (35.9163, 13.3545)
  line L277 (35.9163, 9.6128) -> (35.4163, 9.6128)
  line L278 (37.0206, 13.3545) -> (37.0206, 9.6128)
  line L279 (36.5206, 9.6128) -> (36.5206, 13.3545)
  line L280 (36.5206, 13.3545) -> (37.0206, 13.3545)
  line L281 (37.0206, 9.6128) -> (36.5206, 9.6128)
  line L282 (38.1249, 13.3545) -> (38.1249, 9.6128)
  line L283 (37.6249, 9.6128) -> (37.6249, 13.3545)
  line L284 (37.6249, 13.3545) -> (38.1249, 13.3545)
  line L285 (38.1249, 9.6128) -> (37.6249, 9.6128)
  line L286 (39.2292, 13.3545) -> (39.2292, 9.6128)
  line L287 (38.7292, 9.6128) -> (38.7292, 13.3545)
  line L288 (38.7292, 13.3545) -> (39.2292, 13.3545)
  line L289 (39.2292, 9.6128) -> (38.7292, 9.6128)
  line L290 (40.3334, 13.3545) -> (40.3334, 9.6128)
  line L291 (39.8334, 9.6128) -> (39.8334, 13.3545)
  line L292 (39.8334, 13.3545) -> (40.3334, 13.3545)
  line L293 (40.3334, 9.6128) -> (39.8334, 9.6128)
  line L294 (41.4377, 13.3545) -> (41.4377, 9.6128)
  line L295 (40.9377, 9.6128) -> (40.9377, 13.3545)
  line L296 (40.9377, 13.3545) -> (41.4377, 13.3545)
  line L297 (41.4377, 9.6128) -> (40.9377, 9.6128)
  line L298 (42.542, 13.3545) -> (42.542, 9.6128)
  line L299 (42.042, 9.6128) -> (42.042, 13.3545)
  line L300 (42.042, 13.3545) -> (42.542, 13.3545)
  line L301 (42.542, 9.6128) -> (42.042, 9.6128)
  line L302 (43.6463, 13.3545) -> (43.6463, 9.6128)
  line L303 (43.1463, 9.6128) -> (43.1463, 13.3545)
  line L304 (43.1463, 13.3545) -> (43.6463, 13.3545)
  line L305 (43.6463, 9.6128) -> (43.1463, 9.6128)
  line L306 (44.7506, 13.3545) -> (44.7506, 9.6128)
  line L307 (44.2506, 9.6128) -> (44.2506, 13.3545)
  line L308 (44.2506, 13.3545) -> (44.7506, 13.3545)
  line L309 (44.7506, 9.6128) -> (44.2506, 9.6128)
  line L310 (45.8549, 13.3545) -> (45.8549, 9.6128)
  line L311 (45.3549, 9.6128) -> (45.3549, 13.3545)
  line L312 (45.3549, 13.3545) -> (45.8549, 13.3545)
  line L313 (45.8549, 9.6128) -> (45.3549, 9.6128)
  line L314 (46.9592, 13.3545) -> (46.9592, 9.6128)
  line L315 (46.4592, 9.6128) -> (46.4592, 13.3545)
  line L316 (46.4592, 13.3545) -> (46.9592, 13.3545)
  line L317 (46.9592, 9.6128) -> (46.4592, 9.6128)
  line L318 (48.0634, 13.3545) -> (48.0634, 9.6128)
  line L319 (47.5634, 9.6128) -> (47.5634, 13.3545)
  line L320 (47.5634, 13.3545) -> (48.0634, 13.3545)
  line L321 (48.0634, 9.6128) -> (47.5634, 9.6128)
  line L322 (49.1677, 13.3545) -> (49.1677, 9.6128)
  line L323 (48.6677, 9.6128) -> (48.6677, 13.3545)
  line L324 (48.6677, 13.3545) -> (49.1677, 13.3545)
  line L325 (49.1677, 9.6128) -> (48.6677, 9.6128)
  line L326 (50.272, 13.3545) -> (50.272, 9.6128)
  line L327 (49.772, 9.6128) -> (49.772, 13.3545)
  line L328 (49.772, 13.3545) -> (50.272, 13.3545)
  line L329 (50.272, 9.6128) -> (49.772, 9.6128)
  line L330 (51.3763, 13.3545) -> (51.3763, 9.6128)
  line L331 (50.8763, 9.6128) -> (50.8763, 13.3545)
  line L332 (50.8763, 13.3545) -> (51.3763, 13.3545)
  line L333 (51.3763, 9.6128) -> (50.8763, 9.6128)
  line L334 (52.4806, 13.3545) -> (52.4806, 9.6128)
  line L335 (51.9806, 9.6128) -> (51.9806, 13.3545)
  line L336 (51.9806, 13.3545) -> (52.4806, 13.3545)
  line L337 (52.4806, 9.6128) -> (51.9806, 9.6128)
  line L338 (53.5849, 13.3545) -> (53.5849, 9.6128)
  line L339 (53.0849, 9.6128) -> (53.0849, 13.3545)
  line L340 (53.0849, 13.3545) -> (53.5849, 13.3545)
  line L341 (53.5849, 9.6128) -> (53.0849, 9.6128)
  line L342 (54.6892, 13.3545) -> (54.6892, 9.6128)
  line L343 (54.1892, 9.6128) -> (54.1892, 13.3545)
  line L344 (54.1892, 13.3545) -> (54.6892, 13.3545)
  line L345 (54.6892, 9.6128) -> (54.1892, 9.6128)
  line L346 (55.7934, 13.3545) -> (55.7934, 9.6128)
  line L347 (55.2934, 9.6128) -> (55.2934, 13.3545)
  line L348 (55.2934, 13.3545) -> (55.7934, 13.3545)
  line L349 (55.7934, 9.6128) -> (55.2934, 9.6128)
  line L350 (56.8977, 13.3545) -> (56.8977, 9.6128)
  line L351 (56.3977, 9.6128) -> (56.3977, 13.3545)
  line L352 (56.3977, 13.3545) -> (56.8977, 13.3545)
  line L353 (56.8977, 9.6128) -> (56.3977, 9.6128)
  line L354 (58.002, 13.3545) -> (58.002, 9.6128)
  line L355 (57.502, 9.6128) -> (57.502, 13.3545)
  line L356 (57.502, 13.3545) -> (58.002, 13.3545)
  line L357 (58.002, 9.6128) -> (57.502, 9.6128)
  line L358 (59.1063, 13.3545) -> (59.1063, 9.6128)
  line L359 (58.6063, 9.6128) -> (58.6063, 13.3545)
  line L360 (58.6063, 13.3545) -> (59.1063, 13.3545)
  line L361 (59.1063, 9.6128) -> (58.6063, 9.6128)
  line L362 (60.2106, 13.3545) -> (60.2106, 9.6128)
  line L363 (59.7106, 9.6128) -> (59.7106, 13.3545)
  line L364 (59.7106, 13.3545) -> (60.2106, 13.3545)
  line L365 (60.2106, 9.6128) -> (59.7106, 9.6128)
  line L366 (61.3149, 13.3545) -> (61.3149, 9.6128)
  line L367 (60.8149, 9.6128) -> (60.8149, 13.3545)
  line L368 (60.8149, 13.3545) -> (61.3149, 13.3545)
  line L369 (61.3149, 9.6128) -> (60.8149, 9.6128)
  line L370 (62.4192, 13.3545) -> (62.4192, 9.6128)
  line L371 (61.9192, 9.6128) -> (61.9192, 13.3545)
  line L372 (61.9192, 13.3545) -> (62.4192, 13.3545)
  line L373 (62.4192, 9.6128) -> (61.9192, 9.6128)
  line L374 (63.5234, 13.3545) -> (63.5234, 9.6128)
  line L375 (63.0234, 9.6128) -> (63.0234, 13.3545)
  line L376 (63.0234, 13.3545) -> (63.5234, 13.3545)
  line L377 (63.5234, 9.6128) -> (63.0234, 9.6128)
  dimension "d20" = 2
  dimension "d37" = 0.5
  dimension "d40" = 32
  dimension "d41" = 0
  dimension "d48" = 0.5
  dimension "d51" = 29.8
  dimension "d52" = 0
  dimension "d57" = 30.92
  dimension "d58" = 0
  constraint horizontal L6
  constraint vertical L7
  constraint horizontal L8
  constraint vertical L9
  constraint coincident L1.end L2.start
  constraint coincident L4.end L5.start
  constraint horizontal L10
  constraint vertical L11
  constraint horizontal L12
  constraint vertical L13
  constraint coincident L6 L10.start
  constraint horizontal L14
  constraint vertical L15
  constraint horizontal L16
  constraint vertical L17
  constraint coincident L6 L14.start
  constraint horizontal L18
  constraint vertical L19
  constraint horizontal L20
  constraint vertical L21
  constraint midpoint L17 L18.start
  constraint horizontal L22
  constraint vertical L23
  constraint horizontal L24
  constraint vertical L25
  constraint horizontal L26
  constraint vertical L27
  constraint horizontal L28
  constraint vertical L29
  constraint horizontal L146
  constraint vertical L147
  constraint horizontal L148
  constraint vertical L149
  constraint horizontal L150
  constraint vertical L151
  constraint horizontal L152
  constraint vertical L153
  constraint horizontal L262
  constraint vertical L263
  constraint horizontal L264
  constraint vertical L265
  measures "d20" distance of L18.start L20.end
  measures "d37" distance of L26.start L26.end
  measures "d48" distance of L146.start L146.end
extrude "Extrude9" cut sketch "Sketch3" against normal blind 3 contours L1 L2 L6 L7 L8 L13 L14 L19 L20 bodies 1
extrude "Extrude10" cut sketch "Sketch3" against normal blind 6 contours L1 L2 L6 L7 L8 L13 L14 L19 L20 | L6 L14 L15 L16 L17 L18 L19 bodies 1
extrude "Extrude11" add sketch "Sketch3" along normal blind 3 separate body contours L6 L10 L14 L17 L18 L19 L21 makes body 8